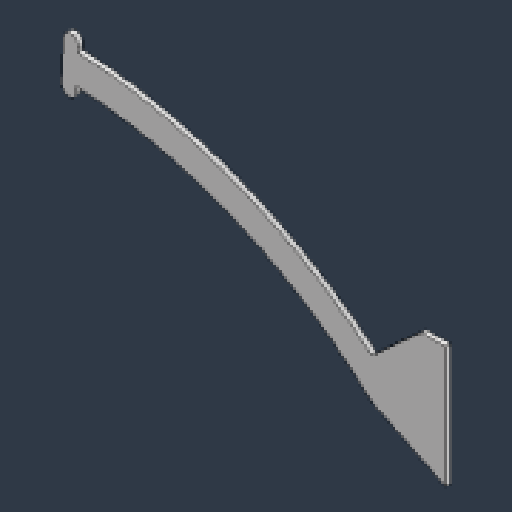
# Autodesk Inventor part: PLATE,SIDE,RACK,INTAKE
Saved by Autodesk Inventor 2026 (Build 300175050, 175E)
## iProperties
Created: 2026-04-12
Part Number: PLATE,SIDE,RACK,INTAKE
Material: Generic
Document SubType Name: Modeling
Designer: Jthib
Mass: 173.039 g
Surface Area: 628.511 cm^2
Volume: 173.039 cm^3
Density: 1 g/cm^3
Appearance: Default
Author: Jthib
Autodesk Inventor part; units mm, degrees
ref_plane "YZ Plane" through (0, 0, 0) normal (1, 0, 0) x (0, 1, 0)
ref_plane "XZ Plane" through (0, 0, 0) normal (0, 1, 0) x (-1, 0, 0)
ref_plane "XY Plane" through (0, 0, 0) normal (0, 0, 1) x (1, 0, 0)
sketch "Sketch1" plane through (0, 0, 0) normal (0, 0, 1) x (1, 0, 0)
  arc A0 (402.7957, 429.3353) -> (29.7943, 587.9503) centre (0, 0) ccw
  arc A1 (428.864, 457.1212) -> (31.7225, 626.0014) centre (0, 0) ccw
  line L0 (31.7225, 626.0014) -> (32.0439, 632.3433)
  arc A2 (32.0439, 632.3433) -> (13.0183, 633.3074) centre (22.5311, 632.8254) ccw
  line L1 (13.0183, 633.3074) -> (10.4473, 582.5725)
  arc A3 (10.4473, 582.5725) -> (29.4729, 581.6084) centre (19.9601, 582.0905) ccw
  line L2 (29.4729, 581.6084) -> (29.7943, 587.9503)
  line L3 (402.7957, 480.2497) -> (464.9618, 536.5258)
  line L4 (464.9618, 536.5258) -> (496.0072, 536.5258)
  line L5 (496.0072, 536.5258) -> (496.0072, 383.2245)
  line L6 (496.0072, 383.2245) -> (402.7957, 429.3353)
  point P0 (0, 0)
  dimension "d0" = 588.7047
  dimension "d1" = 38.1
  dimension "d2" = 9.525
  dimension "d3" = 50.8
  constraints: 14 end point, 9 point on circle, 4 centre point, 4 tangent, 2 collinear, 2 line through centre, 1 coincident, 1 horizontal, 1 parallel, 1 perpendicular
  measures "d0" radius of A0
  measures "d1" radial gap between concentric circles of A0 A1
  measures "d2" radius of A2
  measures "d3" distance of L1.start L1.end
extrude "Extrusion1" add sketch "Sketch1" along normal blind 6.35
body "Solid1"
